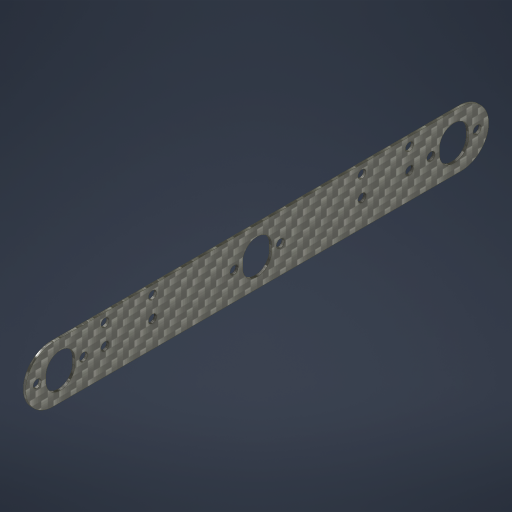
# Autodesk Inventor part: Leg_Loadpipe_Plate_Inner
Saved by Autodesk Inventor 2024 (Build 280153000, 153)
## iProperties
Created: 2023-06-16
Part Number: Leg_Loadpipe_Plate_Inner
Material: CFRP
Document SubType Name: Modeling
Designer: dzw04
Density: 1.43 g/cm^3
Appearance: Carbon Fiber 1
Author: dzw04
Autodesk Inventor part; units mm, degrees
ref_plane "YZ Plane" through (0, 0, 0) normal (1, 0, 0) x (0, 1, 0)
ref_plane "XZ Plane" through (0, 0, 0) normal (0, 1, 0) x (-1, 0, 0)
ref_plane "XY Plane" through (0, 0, 0) normal (0, 0, 1) x (1, 0, 0)
sketch "Sketch1" plane through (0, 0, 0) normal (1, 0, 0) x (0, 1, 0)
  line L0 (-1.25, 6.25) -> (1.25, 6.25)
  arc A0 (1.25, -6.25) -> (1.25, 6.25) centre (1.25, 0) ccw
  line L1 (1.25, -6.25) -> (-1.25, -6.25)
  arc A1 (-1.25, 6.25) -> (-1.25, -6.25) centre (-1.25, 0) ccw
  circle A2 centre (0, -10) radius 1.75
  circle A3 centre (0, 10) radius 1.75
  circle A4 centre (8.25, 45.25) radius 1.75
  circle A5 centre (8.25, 65.75) radius 1.75
  line L2 (-1.25, 91.25) -> (1.25, 91.25)
  arc A6 (1.25, 78.75) -> (1.25, 91.25) centre (1.25, 85) ccw
  line L3 (1.25, 78.75) -> (-1.25, 78.75)
  arc A7 (-1.25, 91.25) -> (-1.25, 78.75) centre (-1.25, 85) ccw
  circle A8 centre (0, 75) radius 1.75
  circle A9 centre (0, 95) radius 1.75
  line L4 (-1.25, -91.25) -> (1.25, -91.25)
  arc A10 (1.25, -91.25) -> (1.25, -78.75) centre (1.25, -85) ccw
  line L5 (1.25, -78.75) -> (-1.25, -78.75)
  arc A11 (-1.25, -78.75) -> (-1.25, -91.25) centre (-1.25, -85) ccw
  circle A12 centre (0, -75) radius 1.75
  circle A13 centre (0, -95) radius 1.75
  circle A14 centre (-0.614, 45.25) radius 1.75
  circle A15 centre (-0.614, 65.75) radius 1.75
  circle A16 centre (8.25, -45.25) radius 1.75
  circle A17 centre (8.25, -65.75) radius 1.75
  circle A18 centre (-0.614, -45.25) radius 1.75
  circle A19 centre (-0.614, -65.75) radius 1.75
  arc A20 (12, 88) -> (-12, 88) centre (0, 88) ccw
  line L6 (12, 88) -> (12, -88)
  arc A21 (-12, -88) -> (12, -88) centre (0, -88) ccw
  line L7 (-12, -88) -> (-12, 88)
  point P0 (0, 0)
  point P1 (0, 0)
  point P2 (-12, -88)
  point P3 (12, 88)
  point P4 (-12, 88)
  point P5 (1.25, -78.75)
  point P6 (1.25, 78.75)
  point P7 (-1.25, 78.75)
  point P8 (1.25, -6.25)
  point P9 (-1.25, -6.25)
  constraints: 22 centre point, 16 end point, 16 point on circle
extrude "Extrusion1" add sketch "Sketch1" along normal blind 1
body "Solid1"
